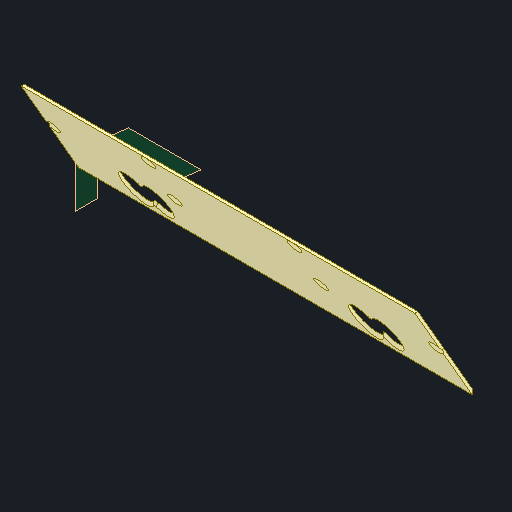
# Autodesk Inventor part: front
Saved by Autodesk Inventor 2023 (Build 270158000, 158)
## iProperties
Created: 2024-05-26
Part Number: front
Material: Nylon 6
Document SubType Name: Modeling
Designer: szymo
Density: 1.12 g/cm^3
Appearance: Nylon 6
Mass: 10.9722 g
Surface Area: 175.007 cm^2
Volume: 9.7966 cm^3
TOTAL MASS: 0.0
Author: szymo
Autodesk Inventor part; units mm, degrees
ref_plane "YZ Plane" through (0, 0, 0) normal (1, 0, 0) x (0, 1, 0)
ref_plane "XZ Plane" through (0, 0, 0) normal (0, 1, 0) x (-1, 0, 0)
ref_plane "XY Plane" through (0, 0, 0) normal (0, 0, 1) x (1, 0, 0)
ref_plane "Work Plane1" through (-178, 0.5, -3.5) normal (-1, 0, 0) x (0, 0, 1)
sketch "Sketch1" plane through (-178, 0.5, -3.5) normal (-1, 0, 0) x (0, 0, 1)
  line L0 (3.5, 3.5) -> (-1, 3.5) projected
  line L1 (-1, 3.5) -> (-1, -0.5) projected
  line L2 (-1, -0.5) -> (-4.5, -0.5) projected
  line L3 (-4.5, -0.5) -> (-4.5, -14.5) projected
  line L4 (-4.5, -14.5) -> (4.5, -0.5) projected
  line L5 (4.5, -0.5) -> (3.5, -0.5) projected
  line L6 (3.5, -0.5) -> (3.5, 3.5) projected
  circle A0 centre (8.5, 158.5) radius 3 projected
  circle A1 centre (8.5, 158.5) radius 25
  circle A2 centre (13, 116) radius 15 projected
  line L7 (3.5, 3.5) -> (28, 45.9352)
  line L8 (3.5, 1.1) -> (29.3856, 45.9352)
  line L9 (29.3856, 45.9352) -> (28, 45.9352)
  line L10 (28, 45.9352) -> (28, 130) projected
  dimension "d0" = 50
  dimension "d1" = 30
  dimension "d3" = 1.2
  dimension "d4" = 2.4
  dimension "d5" = 1.3856
  constraints: 6 end point, 2 point on line, 1 centre point, 1 coincident, 1 horizontal, 1 parallel
  measures "d0" diameter of A1
  measures "d1" angle of L7 L6
  measures "d3" distance between parallel lines of L8 L7
  measures "d4" distance of L8.start L0.start
  measures "d5" distance of L7.end L8.end
ref_plane "Work Plane2" through (0, -14, -8) normal (1, 0, 0) x (0, 1, 0)
extrude "Extrusion1" add sketch "Sketch1" against normal up to surface (178 mm away) contours L7 L9 L8 L6
ref_plane "Work Plane3" through (-141.1151, 26.996, 4.2847) normal (0, -0.9925462, 0.1218693) x (1, 0, 0)
sketch "Sketch3" plane through (-141.1151, 26.996, 4.2847) normal (0, -0.9925462, 0.1218693) x (1, 0, 0)
  line L0 (89.3087, 5.4518) -> (89.3087, -5.4534)
  spline S0 degree 3 poles (89.3087, -5.4534) (89.308, -5.5772) (89.3587, -5.6989) (89.4451, -5.7853) (89.4649, -5.8051) (89.4865, -5.823) (89.5096, -5.8388) (89.529, -5.8521) (89.5494, -5.864) (89.5707, -5.8743) (89.5866, -5.882) (89.603, -5.8889) (89.6197, -5.8948) (89.6699, -5.9125) (89.7231, -5.9218) (89.7769, -5.9215) knots 0 0 0 0 0.5 0.5 0.5 0.614375 0.614375 0.614375 0.710781 0.710781 0.710781 0.783086 0.783086 0.783086 1 1 1 1
  line L1 (89.7769, -5.9215) -> (118.6836, -5.9215)
  spline S1 degree 3 poles (118.6836, -5.9215) (118.8077, -5.9222) (118.9296, -5.8713) (119.1025, -5.6977) (119.1524, -5.5758) (119.1517, -5.4518) knots 0 0 0 0 0.5 0.5 1 1 1 1
  line L2 (119.1517, -5.4518) -> (119.1517, 5.4534)
  spline S2 degree 3 poles (119.1517, 5.4534) (119.1524, 5.5775) (119.1015, 5.6994) (118.9279, 5.8723) (118.806, 5.9222) (118.682, 5.9215) knots 0 0 0 0 0.5 0.5 1 1 1 1
  line L3 (118.682, 5.9215) -> (89.7769, 5.9215)
  spline S3 degree 3 poles (89.7769, 5.9215) (89.6527, 5.9222) (89.5308, 5.8713) (89.3579, 5.6977) (89.308, 5.5758) (89.3087, 5.4518) knots 0 0 0 0 0.5 0.5 1 1 1 1
  circle A0 centre (90.8511, -4.3791) radius 0.5
  circle A1 centre (90.8511, 4.3791) radius 0.5
  circle A2 centre (117.6093, 4.3791) radius 0.5
  circle A3 centre (117.6093, -4.3791) radius 0.5
  arc A4 (104.4919, -1.4512) -> (104.4113, -1.5218) centre (104.5073, -1.55) ccw
  arc A5 (104.4113, 1.5218) -> (104.4113, -1.5218) centre (99.2302, 0) ccw
  arc A6 (104.4113, 1.5218) -> (104.4919, 1.4512) centre (104.5073, 1.55) ccw
  arc A7 (104.4919, 1.4512) -> (104.5716, 1.519) centre (104.4765, 1.55) ccw
  arc A8 (104.5716, -1.519) -> (104.5716, 1.519) centre (109.2302, 0) ccw
  arc A9 (104.5716, -1.519) -> (104.4919, -1.4512) centre (104.4765, -1.55) ccw
  line L4 (-14.6217, 5.4518) -> (-14.6217, -5.4534)
  spline S4 degree 3 poles (-14.6217, -5.4534) (-14.6224, -5.5772) (-14.5717, -5.6989) (-14.4853, -5.7853) (-14.4655, -5.8051) (-14.4439, -5.823) (-14.4208, -5.8388) (-14.4014, -5.8521) (-14.3809, -5.864) (-14.3597, -5.8743) (-14.3438, -5.882) (-14.3274, -5.8889) (-14.3107, -5.8948) (-14.2605, -5.9125) (-14.2073, -5.9218) (-14.1535, -5.9215) knots 0 0 0 0 0.5 0.5 0.5 0.614375 0.614375 0.614375 0.710781 0.710781 0.710781 0.783086 0.783086 0.783086 1 1 1 1
  line L5 (-14.1535, -5.9215) -> (14.7532, -5.9215)
  spline S5 degree 3 poles (14.7532, -5.9215) (14.8773, -5.9222) (14.9992, -5.8713) (15.1721, -5.6977) (15.222, -5.5758) (15.2213, -5.4518) knots 0 0 0 0 0.5 0.5 1 1 1 1
  line L6 (15.2213, -5.4518) -> (15.2213, 5.4534)
  spline S6 degree 3 poles (15.2213, 5.4534) (15.222, 5.5775) (15.1711, 5.6994) (14.9975, 5.8723) (14.8757, 5.9222) (14.7516, 5.9215) knots 0 0 0 0 0.5 0.5 1 1 1 1
  line L7 (14.7516, 5.9215) -> (-14.1535, 5.9215)
  spline S7 degree 3 poles (-14.1535, 5.9215) (-14.2776, 5.9222) (-14.3996, 5.8713) (-14.5725, 5.6977) (-14.6224, 5.5758) (-14.6217, 5.4518) knots 0 0 0 0 0.5 0.5 1 1 1 1
  circle A10 centre (-13.0792, -4.3791) radius 0.5
  circle A11 centre (-13.0792, 4.3791) radius 0.5
  circle A12 centre (13.6789, 4.3791) radius 0.5
  circle A13 centre (13.6789, -4.3791) radius 0.5
  arc A14 (0.5615, -1.4512) -> (0.4809, -1.5218) centre (0.5769, -1.55) ccw
  arc A15 (0.4809, 1.5218) -> (0.4809, -1.5218) centre (-4.7002, 0) ccw
  arc A16 (0.4809, 1.5218) -> (0.5615, 1.4512) centre (0.5769, 1.55) ccw
  arc A17 (0.5615, 1.4512) -> (0.6412, 1.519) centre (0.5461, 1.55) ccw
  arc A18 (0.6412, -1.519) -> (0.6412, 1.519) centre (5.2998, 0) ccw
  arc A19 (0.6412, -1.519) -> (0.5615, -1.4512) centre (0.5461, -1.55) ccw
  circle A20 centre (99.2302, 0) radius 5.4
  circle A21 centre (109.2302, 0) radius 4.9
  circle A22 centre (-4.7002, 0) radius 5.4
  circle A23 centre (5.2998, 0) radius 4.9
  arc A24 (0.5923, 3.0331) -> (0.5923, -3.0331) centre (-4.7002, 0) ccw
  arc A25 (0.5923, -3.0331) -> (0.5923, 3.0331) centre (5.2998, 0) ccw
  arc A26 (104.5227, -3.0331) -> (104.5227, 3.0331) centre (109.2302, 0) ccw
  arc A27 (104.5227, 3.0331) -> (104.5227, -3.0331) centre (99.2302, 0) ccw
  point P0 (141.1151, -7.5427)
  point P1 (104.4877, 1.2324)
  point P2 (104.4113, 1.5218)
  point P3 (104.4113, -1.5218)
  point P4 (104.4877, -1.2324)
  point P5 (104.5716, -1.519)
  point P6 (104.5716, 1.519)
  point P7 (0.5573, 1.2324)
  point P8 (0.4809, 1.5218)
  point P9 (0.4809, -1.5218)
  point P10 (0.5573, -1.2324)
  point P11 (0.6412, -1.519)
  point P12 (0.6412, 1.519)
  dimension "d19" = 0.7
  dimension "d20" = 0.7
  constraints: 8 centre point, 8 point on circle, 4 coincident, 4 concentric, 2 other
  measures "d19" radial gap between concentric circles of A18 A25
  measures "d20" radial gap between concentric circles of A5 A27
extrude "Extrusion2" cut sketch "Sketch3" along normal up to next contours A27 L3 | L3 A27 A26 L1 | L1 A27 | A4 A20 A21 A9 | A5 A20 A21 | A21 A20 A8 | A6 A7 A21 A20 | A21 A20 | A24 L7 | L7 A24 A25 L5 | L5 A24 | A14 A22 A23 A19 | A15 A22 A23 | A23 A22 A18 | A16 A17 A23 A22 | A23 A22
fillet "Fillet1" radius 1 3 edges at (-140.5228, 17.5277, 8.5031) (-140.5228, 8.7984, 3.4632) (-36.5924, 17.5277, 8.5031)
sketch "Sketch4" plane through (-178, 46.4352, 25.8856) normal (0, -0.5, 0.8660254) x (1, 0, 0)
  circle A0 centre (2.5, -24.0381) radius 1.75 projected
  arc A1 (4, -26.5381) -> (5, -25.5381) centre (4, -25.5381) ccw projected
  line L0 (5, -22.5381) -> (5, -25.5381) projected
  arc A2 (5, -22.5381) -> (4, -21.5381) centre (4, -22.5381) ccw projected
  arc A3 (3, -20.5381) -> (4, -21.5381) centre (4, -20.5381) ccw projected
  line L1 (3, -1.8475) -> (3, -20.5381) projected
  ellipse E0 centre (4, -1.8475) end of major axis (4, -0.6928) minor radius 1 (4, -0.6928) -> (3, -1.8475) ccw projected
  line L2 (0, -0.6928) -> (4, -0.6928) projected
  line L3 (0, -47.3834) -> (0, -0.6928) projected
  line L4 (0, -47.3834) -> (1, -47.3834) projected
  line L5 (1, -43.9193) -> (1, -47.3834) projected
  ellipse E1 centre (4, -43.9193) end of major axis (4, -47.3834) minor radius 3 (3, -40.6533) -> (1, -43.9193) ccw projected
  line L6 (3, -27.5381) -> (3, -40.6533) projected
  arc A4 (4, -26.5381) -> (3, -27.5381) centre (4, -27.5381) ccw projected
  circle A5 centre (175.5, -24.0381) radius 1.75 projected
  arc A6 (173, -25.5381) -> (174, -26.5381) centre (174, -25.5381) ccw projected
  arc A7 (175, -27.5381) -> (174, -26.5381) centre (174, -27.5381) ccw projected
  line L7 (175, -27.5381) -> (175, -40.6533) projected
  ellipse E2 centre (174, -43.9193) end of major axis (174, -47.3834) minor radius 3 (177, -43.9193) -> (175, -40.6533) ccw projected
  line L8 (177, -43.9193) -> (177, -47.3834) projected
  line L9 (178, -47.3834) -> (177, -47.3834) projected
  line L10 (178, -47.3834) -> (178, -0.6928) projected
  line L11 (178, -0.6928) -> (174, -0.6928) projected
  ellipse E3 centre (174, -1.8475) end of major axis (174, -0.6928) minor radius 1 (175, -1.8475) -> (174, -0.6928) ccw projected
  line L12 (175, -1.8475) -> (175, -20.5381) projected
  arc A8 (174, -21.5381) -> (175, -20.5381) centre (174, -20.5381) ccw projected
  arc A9 (174, -21.5381) -> (173, -22.5381) centre (174, -22.5381) ccw projected
  line L13 (173, -22.5381) -> (173, -25.5381) projected
  circle A10 centre (122, -27.1641) radius 1.75 projected
  circle A11 centre (122, -3.1928) radius 1.75 projected
  line L14 (124.5, -0.6928) -> (124.5, -32.7447) projected
  line L15 (124.5, -0.6928) -> (119.5, -0.6928) projected
  line L16 (119.5, -0.6928) -> (119.5, -32.7447) projected
  line L17 (58.5, -0.6928) -> (58.5, -32.7447) projected
  line L18 (53.5, -0.6928) -> (53.5, -32.7447) projected
  line L19 (119.5, -32.7447) -> (124.5, -32.7447) projected
  line L20 (58.5, -32.7447) -> (53.5, -32.7447) projected
  line L21 (53.5, -0.6928) -> (58.5, -0.6928) projected
  circle A12 centre (56, -27.1641) radius 1.75 projected
  circle A13 centre (56, -3.1928) radius 1.75 projected
  point P0 (178, -53.1569)
  point P1 (56, -27.193)
  point P2 (56, -3.2217)
  constraints: 4 coincident, 4 other
hole "Hole2" at (-175.5, 25.6176, 13.8666) at (-122, 22.8854, 12.2891) at (-122, 43.6452, 24.2748) at (-56, 22.9104, 12.3036) at (-56, 43.6702, 24.2892) at (-2.5, 25.6176, 13.8666) direction (0, 0.5, -0.8660254) diameter 2.9 end through all countersink diameter 6 countersink angle 90 clearance for "Countersunk Flat Head Screw ISO 2009/7046" size "M2.5" standard "ISO"
body "Solid1"
